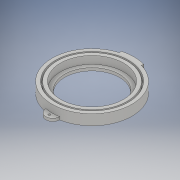
# Autodesk Inventor part: Cap
Saved by Autodesk Inventor 2018 (Build 220112000, 112)
## iProperties
Created: 2017-06-25
Part Number: Cap
Material: Generic
Document SubType Name: Modeling
Designer: Soichi
Density: 1 g/cm^3
Appearance: Default
Author: Soichi
Autodesk Inventor part; units mm, degrees
ref_plane "YZ Plane" through (0, 0, 0) normal (1, 0, 0) x (0, 1, 0)
ref_plane "XZ Plane" through (0, 0, 0) normal (0, 1, 0) x (-1, 0, 0)
ref_plane "XY Plane" through (0, 0, 0) normal (0, 0, 1) x (1, 0, 0)
sketch "Sketch1" plane through (0, 0, 0) normal (0, 0, 1) x (1, 0, 0)
  circle A0 centre (0, 0) radius 57.5
  dimension "d0" = 115
  constraints: 1 centre point, 1 coincident
  measures "d0" diameter of A0
sketch "Sketch2" plane through (0, 0, 0) normal (1, 0, 0) x (0, 1, 0)
  line L0 (57.5, 0) -> (-57.5, 0) construction
  line L1 (-57.5, 0) -> (-57.5, 15)
  line L2 (-57.5, 15) -> (-39.5, 15)
  line L3 (-39.5, 15) -> (-39.5, 11)
  line L4 (-57.5, 0) -> (-52.5, 0)
  line L5 (-52.5, 0) -> (-52.5, 8)
  line L6 (-52.5, 8) -> (-50.42, 8)
  line L7 (-50.42, 8) -> (-50.42, 0)
  line L8 (-50.42, 0) -> (-45.42, 0)
  line L9 (-50.42, 0) -> (-45.42, 0) construction
  line L10 (-45.42, 0) -> (-45.42, 11)
  line L11 (-45.42, 11) -> (-39.5, 11)
  point P0 (0, 0)
  dimension "d1" = 15
  dimension "d3" = 4
  dimension "d4" = 90
  dimension "d5" = 5
  dimension "d6" = 8
  dimension "d7" = 2.08
  dimension "d8" = 5
  dimension "d9" = 0
  dimension "d10" = 90
  dimension "d15" = 13
  constraints: 22 end point, 4 perpendicular, 3 horizontal, 2 point on line, 1 collinear, 1 parallel, 1 vertical
  measures "d1" distance of L0.end L1.end
  measures "d3" distance of L2.end L3.end
  measures "d4" angle of L2 L3
  measures "d5" distance of L0.end L4.end
  measures "d6" distance of L4.end L5.end
  measures "d7" distance of L5.end L6.end
  measures "d8" distance of L7.end L8.end
  measures "d9" distance between parallel lines of L8 L9
  measures "d10" angle of L10 L8
  measures "d15" distance between parallel lines of L3 L5
sweep "Sweep1" add profiles "Sketch2" path "Sketch1"
sketch "Sketch3" plane through (0, 0, 15) normal (0, 0, 1) x (1, 0, 0)
  line L0 (56.5, 10) -> (-56.5, 10) construction
  line L1 (-56.5, 10) -> (-56.5, -10)
  line L2 (-56.5, -10) -> (56.5, -10) construction
  line L3 (56.5, -10) -> (56.5, 10)
  line L4 (56.5, 10) -> (-56.5, -10) construction
  arc A0 (-56.5, 10) -> (-56.5, -10) centre (-56.5, 0) ccw
  circle A1 centre (0, 0) radius 57.5 construction
  line L5 (-55.3308, 15.6447) -> (-55.3308, -15.6447)
  arc A2 (-55.3308, 15.6447) -> (-55.3308, -15.6447) centre (0, 0) ccw
  line L6 (0, 0) -> (-55.3308, -15.6447) construction
  line L7 (-55.3308, -15.6447) -> (-58.3308, -16.4929)
  line L8 (0, 0) -> (-55.3308, 15.6447) construction
  line L9 (-55.3308, 15.6447) -> (-58.3308, 16.4929)
  arc A3 (-58.3308, 16.4929) -> (-58.3308, -16.4929) centre (0, 0) ccw
  arc A4 (58.3308, -16.4929) -> (58.3308, 16.4929) centre (0, 0) ccw
  line L10 (55.3308, -15.6447) -> (58.3308, -16.4929)
  arc A5 (55.3308, -15.6447) -> (55.3308, 15.6447) centre (0, 0) ccw
  line L11 (55.3308, -15.6447) -> (55.3308, 15.6447)
  line L12 (55.3308, 15.6447) -> (58.3308, 16.4929)
  point P0 (-61.5, 0)
  dimension "d17" = 20
  dimension "d18" = 5
  dimension "d19" = 10
  dimension "d31" = 56.5
  dimension "d32" = 31.2894
  dimension "d33" = 3
  dimension "d34" = 3
  dimension "d37" = 360
  constraints: 26 end point, 12 point on circle, 5 centre point, 4 coincident, 2 collinear, 2 midpoint, 2 parallel, 2 point on line, 1 horizontal, 1 perpendicular, 1 vertical, 25 other
  measures "d17" distance of L2.end L0.start
  measures "d18" distance of A0.centre point (-61.5, 0)
  measures "d19" radius of A0
  measures "d31" distance from line of L1 point (0, 0)
  measures "d32" distance of L5.start L5.end
  measures "d33" horizontal distance of L5.end L7.end
  measures "d34" horizontal distance of L5.start L9.end
extrude "Extrusion2" add sketch "Sketch3" against normal blind 4 contours L1 A0 A2 | A2 A0 A3 | A3 A0
hole "Hole1" at (-61.5, 0, 15) direction (0, 0, -1) diameter 3 end through all
extrude "Extrusion3" add sketch "Sketch3" along normal blind 4 and the other way blind 15 contours L10 A5 L12 A4 | L11 A5
extrude "Extrusion4" cut sketch "Sketch3" along normal blind 2.08 contours L11 A5
equation "\"d18\" = 0.5 * d19"
equation "\"d34\" = d33"
body "Solid1"
